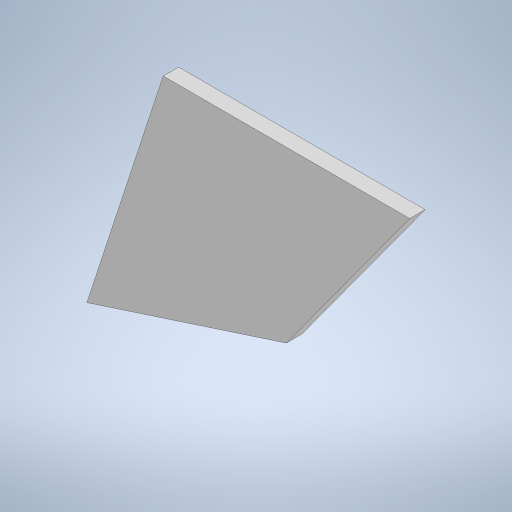
# Autodesk Inventor part: Pieza4
Saved by Autodesk Inventor 2024 (Build 280153000, 153)
## iProperties
Created: 2025-08-12
Part Number: Pieza4
Material: Genérico
Document SubType Name: Modeling
Designer: sergi
Density: 1 g/cm^3
Appearance: Valor por defecto
Author: sergi
Autodesk Inventor part; units mm, degrees
ref_plane "YZ Plane" through (0, 0, 0) normal (1, 0, 0) x (0, 1, 0)
ref_plane "XZ Plane" through (0, 0, 0) normal (0, 1, 0) x (-1, 0, 0)
ref_plane "XY Plane" through (0, 0, 0) normal (0, 0, 1) x (1, 0, 0)
sketch "Boceto1" plane through (0, 0, 0) normal (0, 0, 1) x (1, 0, 0)
  line L0 (-5.101, 7.979) -> (-5.1003, 9.079) projected
  line L1 (-5.1003, 9.079) -> (-5.8995, 9.0795) projected
  line L2 (-5.101, 7.979) -> (-5.8995, 9.0795) projected
  line L3 (-5.8995, 9.0795) -> (-5.1003, 9.079)
  line L4 (-5.101, 7.979) -> (-5.8995, 9.0795)
  line L5 (-5.1003, 9.079) -> (-5.101, 7.979)
  line L6 (-5.1003, 9.079) -> (-4.3011, 9.0785)
  line L7 (-5.101, 7.979) -> (-4.3011, 9.0785)
  point P0 (0, 0)
  constraints: 10 end point, 2 perpendicular, 1 symmetric about line
extrude "Extrusión1" add sketch "Boceto1" along normal blind 0.1
mirror "Simetría1" about plane through (-5.8995, 9.0795, 0) normal (-0.8094085, -0.587246, 0)
